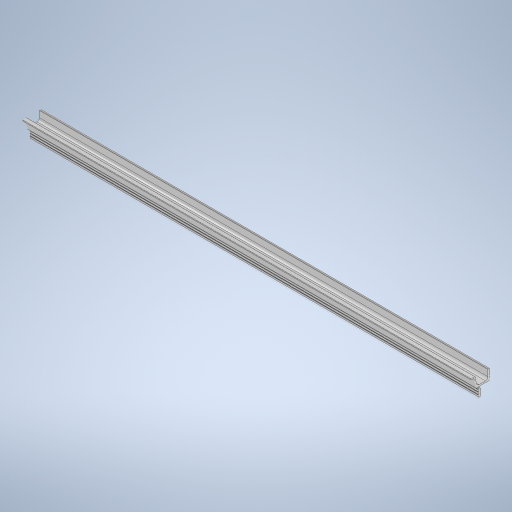
# Autodesk Inventor part: Hafele alu 126_13
Saved by Autodesk Inventor 2024 (Build 280153000, 153)
## iProperties
RuleStatus: InUse
Created: 2019-10-04
Part Number: Hafele alu 126_13
Material: Aluminum 6061
Document SubType Name: Modeling
Designer: RokasM
Density: 2.7 g/cm^3
Appearance: Aluminum - Flat
Author: RokasM
Autodesk Inventor part; units mm, degrees
ref_plane "YZ Plane" through (0, 0, 0) normal (1, 0, 0) x (0, 1, 0)
ref_plane "XZ Plane" through (0, 0, 0) normal (0, 1, 0) x (-1, 0, 0)
ref_plane "XY Plane" through (0, 0, 0) normal (0, 0, 1) x (1, 0, 0)
sketch "Sketch1" plane through (0, 0, 0) normal (1, 0, 0) x (0, 1, 0)
  line L0 (14.5, 11.2) -> (14.5, 0)
  line L1 (14.5, 0) -> (4.3, 0)
  line L2 (4.3, 0) -> (4.3, -2.5)
  line L3 (4.3, -2.5) -> (4.85, -2.5)
  line L4 (4.85, -2.5) -> (4.3, -5)
  line L5 (4.3, -5) -> (4.85, -5)
  line L6 (4.85, -5) -> (4.3, -7.5)
  line L7 (4.3, -7.5) -> (4.85, -7.5)
  line L8 (4.85, -7.5) -> (4.3, -10)
  line L9 (4.3, -10) -> (2.9, -10)
  line L10 (2.9, -10) -> (2.35, -7.5)
  line L11 (2.35, -7.5) -> (2.9, -7.5)
  line L12 (2.9, -7.5) -> (2.35, -5)
  line L13 (2.35, -5) -> (2.9, -5)
  line L14 (2.9, -5) -> (2.35, -2.5)
  line L15 (2.35, -2.5) -> (2.9, -2.5)
  line L16 (2.9, -2.5) -> (2.9, 0)
  line L17 (2.9, 0) -> (0, 0)
  line L18 (0, 0) -> (-2.3, 10)
  line L19 (-2.3, 10) -> (-5.3, 10)
  line L20 (-5.3, 10) -> (-5.3, 11.2)
  line L21 (-5.3, 11.2) -> (-1.1, 11.2)
  line L22 (-1.1, 11.2) -> (1.108, 1.6)
  line L23 (1.108, 1.6) -> (12.8, 1.6)
  line L24 (12.8, 1.6) -> (12.8, 11.2)
  line L25 (12.8, 11.2) -> (14.5, 11.2)
  dimension "d0" = 1.7
  dimension "d1" = 1.2
  dimension "d2" = 4.2
  dimension "d3" = 3
  dimension "d4" = 5.3
  dimension "d6" = 10
  dimension "d7" = 10
  dimension "d8" = 2.5
  dimension "d9" = 7.65
  dimension "d10" = 19.8
  dimension "d11" = 2.5
  dimension "d12" = 0.55
  dimension "d13" = 1.6
  constraints: 52 end point, 8 horizontal, 6 equal length, 5 collinear, 5 parallel, 5 vertical, 4 vertical alignment, 2 coincident
  measures "d0" distance between parallel lines of L0 L24
  measures "d1" distance between parallel lines of L19 L21
  measures "d2" distance of L20.end L21.end
  measures "d3" distance of L18.end L19.end
  measures "d4" distance from line of L17.end L20
  measures "d6" distance between parallel lines of L17 L19
  measures "d7" distance between parallel lines of L9 L1
  measures "d8" distance of L7.end L10.end
  measures "d9" distance from line of L14.end L20
  measures "d10" distance between parallel lines of L0 L20
  measures "d11" distance between parallel lines of L5 L7
  measures "d12" distance of L14.end L15.end
  measures "d13" distance between parallel lines of L1 L23
extrude "01_ex1" add sketch "Sketch1" along normal mid plane 480
fillet "01_fillet1" radius 2.5 2 edges at (0, 12.8, 1.6) (0, 1.108, 1.6)
fillet "01_fillet1" radius 0.3 2 edges at (0, 12.8, 11.2) (0, 14.5, 11.2)
fillet "01_fillet1" radius 0.2 16 edges at (0, -1.1, 11.2) (0, -5.3, 11.2) (0, -5.3, 10) (0, -2.3, 10) (0, 0, 0) (0, 2.9, 0) (0, 2.35, -2.5) (0, 2.35, -5) (0, 2.35, -7.5) (0, 2.9, -10) (0, 4.3, -10) (0, 4.85, -7.5) (0, 4.85, -5) (0, 4.85, -2.5) (0, 4.3, 0) (0, 14.5, 0)
sketch "Sketch2" plane through (0, 0, 0) normal (1, 0, 0) x (0, 1, 0)
  line L0 (4.75, 0) -> (4.75, -11)
  line L1 (4.75, -11) -> (2.45, -11)
  line L2 (2.45, -11) -> (2.45, 0)
  line L3 (3.0608, -10) -> (4.1392, -10) projected
  line L4 (4.5, 0) -> (14.3, 0) projected
  line L5 (2.45, 0) -> (0, 0)
  line L6 (0, 0) -> (-2.2643, 9.8448)
  arc A0 (-2.2643, 9.8448) -> (-2.4592, 10) centre (-2.4592, 9.8) ccw
  line L7 (-2.4592, 10) -> (-5.3, 10)
  line L8 (-5.3, 10) -> (-5.3, 11.2)
  line L9 (-5.3, 11.2) -> (14.5, 11.2)
  line L10 (14.5, 11.2) -> (14.5, 0)
  line L11 (14.5, 0) -> (4.75, 0)
  line L12 (-2.2643, 9.8448) -> (-0.0357, 0.1552) projected
  line L13 (-5.1, 10) -> (-2.4592, 10) projected
  arc A1 (-2.2643, 9.8448) -> (-2.4592, 10) centre (-2.4592, 9.8) ccw projected
  line L14 (-5.3, 11) -> (-5.3, 10.2) projected
  line L15 (-1.2592, 11.2) -> (-5.1, 11.2) projected
  line L16 (14.5, 0.2) -> (14.5, 10.9) projected
  line L17 (0.1592, 0) -> (2.7, 0) projected
  point P0 (0, 0)
  point P1 (3.6, -11)
  point P2 (3.6, -10)
  dimension "d19" = 2.3
  dimension "d20" = 1
  constraints: 20 end point, 7 collinear, 2 midpoint, 2 perpendicular, 2 point on circle, 1 centre point, 1 concentric, 1 parallel, 1 tangent, 1 vertical alignment
  measures "d19" distance between parallel lines of L0 L2
  measures "d20" distance between parallel lines of L1 L3
extrude "02_ex1" add sketch "Sketch2" along normal mid plane 480 separate body
equation "\"d14\" = Length"
equation "\"d21\" = Length"
equation "\"Length\" = 480"
